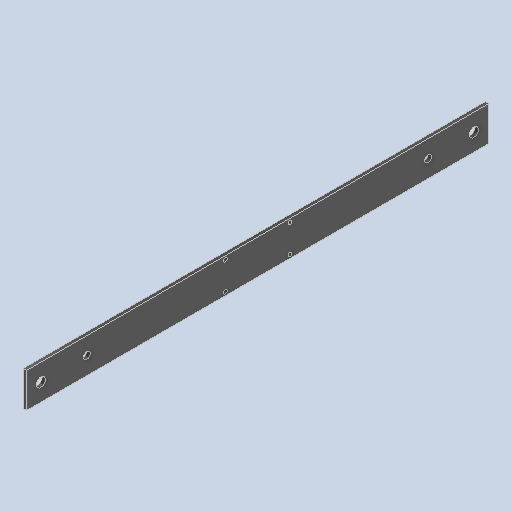
# Autodesk Inventor part: HCMUTE-CDT23-OP_DVCAM
Saved by Autodesk Inventor 2023 (Build 270158000, 158)
## iProperties
Created: 2023-11-14
Part Number: HCMUTE-CDT23-OP_DVCAM
Material: PMMA Plastic
Document SubType Name: Sheet Metal
Designer: havie
Density: 1.188 g/cm^3
Sheet Metal Rule: Default_mm
Appearance: Dark Gray
Author: havie
Autodesk Inventor part; units mm, degrees
ref_plane "YZ Plane" through (0, 0, 0) normal (1, 0, 0) x (0, 1, 0)
ref_plane "XZ Plane" through (0, 0, 0) normal (0, 1, 0) x (-1, 0, 0)
ref_plane "XY Plane" through (0, 0, 0) normal (0, 0, 1) x (1, 0, 0)
sketch "Sketch2" plane through (-1.5, 0, 0) normal (-1, 0, 0) x (0, 0, 1)
  circle A0 centre (177.25, 0.2229) radius 2.55 projected
  circle A1 centre (157.25, 0.2229) radius 2.55 projected
  point P0 (0, 0)
sketch "Sketch1" plane through (0, 0, 0) normal (1, 0, 0) x (0, 1, 0)
  line L0 (15, 200) -> (-15, 200)
  line L1 (-15, 200) -> (-15, -200)
  line L2 (-15, -200) -> (15, -200)
  line L3 (15, -200) -> (15, 200)
  line L4 (15, 200) -> (-15, -200) construction
  line L5 (-15, 200) -> (15, -200) construction
  point P0 (0, 0)
  point P1 (0, 0)
  dimension "d0" = 400
  dimension "d1" = 30
  measures "d0" distance of L2.end L0.start
  measures "d1" distance of L0.start L0.end
extrude "Plate1" add sketch "Sketch1" along normal mid plane 3
sketch "Sketch3" plane through (-1.5, 0, 0) normal (-1, 0, 0) x (0, 0, 1)
  circle A0 centre (187.6, 0) radius 4
  circle A1 centre (147.9, 0) radius 3
  circle A2 centre (-147.4, 0) radius 3
  circle A3 centre (-187.1, 0) radius 4
  line L0 (200, 15) -> (200, -15) projected
  line L1 (-200, -15) -> (-200, 15) projected
  line L2 (200, -15) -> (-200, -15) projected
  point P0 (0, 0)
  dimension "d7" = 12.4
  dimension "d8" = 8
  dimension "d9" = 39.7
  dimension "d10" = 6
  dimension "d22" = 8
  dimension "d23" = 6
  dimension "d24" = 12.9
  dimension "d26" = 15
  dimension "d27" = 39.7
  constraints: 4 centre point, 3 horizontal alignment
  measures "d7" distance from line of L0 A0.centre
  measures "d8" diameter of A0
  measures "d9" distance of A0.centre A1.centre
  measures "d10" diameter of A1
  measures "d22" diameter of A3
  measures "d23" diameter of A2
  measures "d24" distance from line of L1 A3.centre
  measures "d26" distance from line of L2 A3.centre
  measures "d27" distance of A2.centre A3.centre
extrude "Cut2" cut sketch "Sketch3" against normal blind 3
sketch "Sketch4" plane through (1.5, 0, 0) normal (1, 0, 0) x (0, 0, -1)
  line L0 (-200, 15) -> (200, 15) projected
  point P0 (0, 0)
  point P1 (-28, 12)
  point P2 (-28, -12)
  point P3 (28, 12)
  point P4 (28, -12)
  dimension "d11" = 56
  dimension "d12" = 24
  dimension "d13" = 3
  dimension "d14" = 28
  constraints: 2 horizontal alignment, 2 vertical alignment
  measures "d11" distance of point (28, 12) point (-28, 12)
  measures "d12" distance of point (-28, -12) point (-28, 12)
  measures "d13" distance from line of L0 point (-28, 12)
  measures "d14" horizontal distance of point (0, 0) point (-28, 12)
hole "Hole1" at (1.5, 12, 28) at (1.5, -12, 28) at (1.5, 12, -28) at (1.5, -12, -28) direction (-1, 0, 0) diameter 3.242 depth 11.8 tip angle 118 thread size "M4x0.7" class "6H" standard "ISO Metric profile"
equation "\"d27\" = d9"
equation "\"d5\" = Thickness"
equation "\"d2\" = Thickness"
equation "\"BendRadius\" = Thickness"
equation "\"BendReliefWidth\" = Thickness"
equation "\"BendReliefDepth\" = 0.5 * Thickness"
equation "\"CornerReliefSize\" = 4 * Thickness"
equation "\"MinimumRemnant\" = 2 * Thickness"
equation "\"TransitionRadius\" = BendRadius"
equation "\"JacobiRadiusSize\" = BendRadius"
equation "\"GapSize\" = Thickness"
equation "\"Thickness\" = 3"
body "Solid1"
